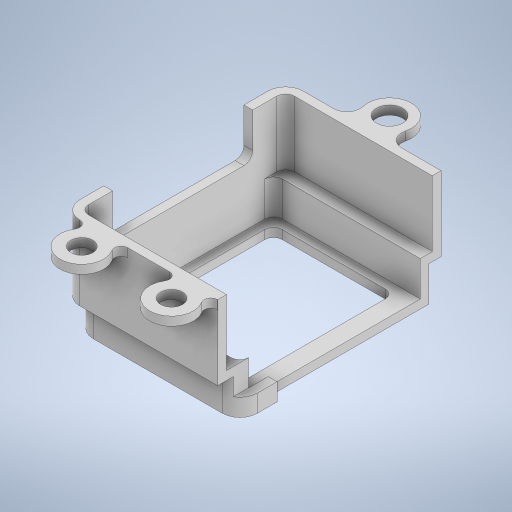
# Autodesk Inventor part: CO-1-01-motorControllersMount
Saved by Autodesk Inventor 2023 (Build 270158000, 158)
## iProperties
Created: 2023-01-24
Part Number: CO-1-01-motorControllersMount
Material: Generic
Document SubType Name: Modeling
Designer: t205b
Density: 1 g/cm^3
Appearance: Default
Author: t205b
Autodesk Inventor part; units mm, degrees
ref_plane "YZ Plane" through (0, 0, 0) normal (1, 0, 0) x (0, 1, 0)
ref_plane "XZ Plane" through (0, 0, 0) normal (0, 1, 0) x (-1, 0, 0)
sketch "Sketch1" plane through (0, 0, 0) normal (0, 1, 0) x (-1, 0, 0)
  arc A0 (31.569, 13.7227) -> (30.069, 12.2227) centre (31.569, 12.2227) ccw
  line L0 (31.569, 13.7227) -> (34.069, 13.7227)
  line L1 (34.069, 13.7227) -> (34.069, 18.9227)
  line L2 (32.069, 20.9227) -> (2.569, 20.9227)
  line L3 (34.069, -13.2773) -> (31.569, -13.2773)
  arc A1 (30.069, -11.7773) -> (31.569, -13.2773) centre (31.569, -11.7773) ccw
  arc A2 (34.069, 18.9227) -> (32.069, 20.9227) centre (32.069, 18.9227) ccw
  arc A3 (34.0195, 22.4149) -> (32.069, 23.9727) centre (32.069, 21.9727) ccw
  line L4 (32.069, 23.9727) -> (-23.931, 23.9727)
  arc A4 (-23.931, 23.9727) -> (-25.931, 21.9727) centre (-23.931, 21.9727) ccw
  line L5 (-25.931, 21.9727) -> (-25.931, -21.0273)
  arc A5 (-25.931, -21.0273) -> (-23.931, -23.0273) centre (-23.931, -21.0273) ccw
  line L6 (-23.931, -23.0273) -> (32.069, -23.0273)
  arc A6 (32.069, -23.0273) -> (33.899, -21.8341) centre (32.069, -21.0273) ccw
  arc A7 (32.069, -20.2773) -> (34.069, -18.2773) centre (32.069, -18.2773) ccw
  line L7 (32.069, -20.2773) -> (0.569, -20.2773)
  line L8 (34.069, -13.2773) -> (34.069, 13.7227)
  line L9 (0.569, -22.2773) -> (0.569, 18.9227)
  line L10 (30.069, -11.7773) -> (30.069, 12.2227)
  line L11 (34.069, -18.2773) -> (34.069, -13.2773)
  line L12 (2.569, 22.9227) -> (32.069, 22.9227)
  line L13 (0.569, -22.2773) -> (32.069, -22.2773)
  arc A8 (32.069, -22.2773) -> (36.069, -18.2773) centre (32.069, -18.2773) ccw
  line L14 (36.069, -18.2773) -> (36.069, 18.9227)
  arc A9 (2.569, 20.9227) -> (0.569, 18.9227) centre (2.569, 18.9227) ccw
  line L15 (-1.431, 14.4227) -> (-1.431, 18.9227)
  arc A10 (2.569, 22.9227) -> (-1.431, 18.9227) centre (2.569, 18.9227) ccw
  arc A11 (36.069, 18.9227) -> (32.069, 22.9227) centre (32.069, 18.9227) ccw
  line L16 (-1.431, 14.4227) -> (0.569, 14.4227)
  point P0 (0.569, 20.9227)
  dimension "d8" = 2
  dimension "d9" = 2
  dimension "d66" = 2
  dimension "d67" = 2
  dimension "d68" = 4.5
  dimension "d69" = 4
  constraints: 35 end point, 27 point on circle, 12 centre point, 8 vertical, 6 horizontal, 4 point on line, 3 tangent, 2 perpendicular, 1 collinear, 9 other
  measures "d8" distance between parallel lines of L2 L12
  measures "d9" distance between parallel lines of L7 L13
  measures "d66" radius of A9
  measures "d67" radial gap between concentric circles of A9 A10
  measures "d68" distance of L15.start L15.end
  measures "d69" radius of A11
extrude "Extrusion3" add sketch "Sketch1" against normal blind 2 contours L0 L8 L3 A1 L10 A0 | A0 L10 A1 L3 L11 A7 L7 L9 A9 L2 A2 L1 L0 | L1 A2 L2 A9 L9 L16 L15 A10 L12 A11 L14 A8 L13 L7 A7 L11 L8
ref_plane "Work Plane1" through (0, 8, 0) normal (0, 1, 0) x (1, 0, 0)
extrude "Extrusion4" add sketch "Sketch1" along normal blind 8 contours L1 A2 L2 A9 L9 L16 L15 A10 L12 A11 L14 A8 L13 L7 A7 L11 L8
sketch "Sketch2" plane through (0, 8, 0) normal (0, 1, 0) x (1, 0, 0)
  line L0 (23.931, 23.0273) -> (-32.069, 23.0273) projected
  arc A0 (-32.069, 23.0273) -> (-33.899, 21.8341) centre (-32.069, 21.0273) ccw projected
  line L1 (-32.069, -23.9727) -> (23.931, -23.9727) projected
  arc A1 (-34.0195, -22.4149) -> (-32.069, -23.9727) centre (-32.069, -21.9727) ccw projected
  arc A2 (-32.069, 23.0273) -> (-34.069, 21.0273) centre (-32.069, 21.0273) ccw
  arc A3 (-34.069, -21.9727) -> (-32.069, -23.9727) centre (-32.069, -21.9727) ccw
  line L2 (-34.069, 18.2773) -> (-34.069, 13.2773) projected
  line L3 (-34.069, 13.2773) -> (-34.069, -13.7227) projected
  line L4 (-34.069, -13.7227) -> (-34.069, -18.9227) projected
  line L5 (-34.069, -21.9727) -> (-34.069, 21.0273)
  arc A4 (-32.069, 25.0273) -> (-36.069, 21.0273) centre (-32.069, 21.0273) ccw
  line L6 (-0.569, 25.0273) -> (-32.069, 25.0273)
  line L7 (-0.569, -25.9727) -> (-32.069, -25.9727)
  line L8 (-0.569, -23.9727) -> (-0.569, -25.9727)
  line L9 (-0.569, 20.2773) -> (-0.569, 25.0273)
  line L10 (-0.569, 22.2773) -> (-0.569, 22.2773) projected
  line L11 (-32.069, 23.0273) -> (-0.569, 23.0273)
  line L12 (-32.069, -23.9727) -> (-0.569, -23.9727)
  line L13 (-32.069, -20.9227) -> (-2.569, -20.9227) projected
  line L14 (-0.569, -14.4227) -> (-0.569, 20.2773) projected
  line L15 (-0.569, 20.2773) -> (-32.069, 20.2773) projected
  arc A5 (-32.069, 20.2773) -> (-34.069, 18.2773) centre (-32.069, 18.2773) ccw projected
  line L16 (-34.069, 18.2773) -> (-34.069, -18.9227) projected
  arc A6 (-34.069, -18.9227) -> (-32.069, -20.9227) centre (-32.069, -18.9227) ccw projected
  line L17 (-32.069, 22.2773) -> (-0.569, 22.2773) projected
  line L18 (-0.569, 22.2773) -> (-0.569, 22.2773)
  arc A7 (-2.569, -20.9227) -> (-0.569, -18.9227) centre (-2.569, -18.9227) ccw projected
  line L19 (-0.569, -18.9227) -> (-0.569, -14.4227) projected
  line L20 (-0.569, -23.9727) -> (-0.569, -18.9227)
  line L21 (-36.069, 21.0273) -> (-36.069, -21.9727)
  arc A8 (-36.069, -21.9727) -> (-32.069, -25.9727) centre (-32.069, -21.9727) ccw
  point P0 (0, 0)
  point P1 (-32.069, 25.0273)
  dimension "d19" = 2
  dimension "d20" = 2
  dimension "d21" = 31.5
  dimension "d22" = 31.5
  dimension "d23" = 31.5
  constraints: 22 end point, 10 point on circle, 6 point on line, 4 centre point, 4 perpendicular, 3 tangent, 2 coincident, 2 vertical, 1 concentric, 1 horizontal, 1 parallel, 1 vertical alignment, 1 other
  measures "d19" distance between parallel lines of L0 L6
  measures "d20" distance between parallel lines of L1 L7
  measures "d21" distance of L7.start L7.end
  measures "d22" distance of L1.start L8.start
  measures "d23" distance of L6.start L6.end
extrude "Extrusion7" add sketch "Sketch2" against normal blind 2 contours L9 L15 A5 L5 A2 A0 L0 | L0 A0 A2 L5 L2 L3 L4 A3 A1 L1 L8 L7 A8 L21 A4 L6 L9 | L20 L1 A1 A3 L5 A6 L13 A7
extrude "Extrusion8" add sketch "Sketch2" along normal blind 15 contours L0 A0 A2 L5 L2 L3 L4 A3 A1 L1 L8 L7 A8 L21 A4 L6 L9
sketch "Sketch5" plane through (0, 23, 0) normal (0, 1, 0) x (1, 0, 0)
  circle A0 centre (-17.319, 30.0273) radius 5
  circle A1 centre (-17.319, 30.0273) radius 3
  arc A2 (-12.4777, 28.7773) -> (-9.573, 25.0273) centre (-9.573, 28.0273) ccw
  arc A3 (-25.0649, 25.0273) -> (-22.1602, 28.7773) centre (-25.0649, 28.0273) ccw
  line L0 (-0.569, 23.0273) -> (-0.569, 25.0273) projected
  circle A4 centre (-6.0917, -30.9727) radius 5
  circle A5 centre (-6.0917, -30.9727) radius 2.5
  arc A6 (-10.305, -28.2804) -> (-11.569, -25.9727) centre (-11.569, -27.4727) ccw
  arc A7 (-0.6145, -25.9727) -> (-1.8785, -28.2804) centre (-0.6145, -27.4727) ccw
  circle A8 centre (-26.5917, -30.9727) radius 5
  circle A9 centre (-26.5917, -30.9727) radius 2.5
  arc A10 (-30.805, -28.2804) -> (-32.069, -25.9727) centre (-32.069, -27.4727) ccw
  arc A11 (-21.1145, -25.9727) -> (-22.3785, -28.2804) centre (-21.1145, -27.4727) ccw
  line L1 (-0.569, -25.9727) -> (-0.569, -23.9727) projected
  line L2 (-0.569, 25.0273) -> (-32.069, 25.0273) projected
  line L3 (-32.069, -25.9727) -> (-0.569, -25.9727) projected
  point P0 (0, 0)
  point P1 (1.0185, -24.3852)
  point P2 (-26.5917, -25.9727)
  point P3 (-6.0917, -25.9727)
  point P4 (-17.319, 25.0273)
  dimension "d34" = 10
  dimension "d35" = 6
  dimension "d38" = 3
  dimension "d39" = 3
  dimension "d40" = 10
  dimension "d41" = 5
  dimension "d42" = 3
  dimension "d43" = 3
  dimension "d44" = 10
  dimension "d45" = 5
  dimension "d46" = 3
  dimension "d47" = 3
  dimension "d49" = 20.5
  constraints: 18 point on circle, 12 centre point, 6 tangent, 3 coincident
  measures "d34" diameter of A0
  measures "d35" diameter of A1
  measures "d38" radius of A3
  measures "d39" radius of A2
  measures "d40" diameter of A4
  measures "d41" diameter of A5
  measures "d42" diameter of A6
  measures "d43" diameter of A7
  measures "d44" diameter of A8
  measures "d45" diameter of A9
  measures "d46" diameter of A10
  measures "d47" diameter of A11
  measures "d49" distance of A4.centre A8.centre
extrude "Extrusion10" add sketch "Sketch5" against normal blind 2
sketch "Sketch6" plane through (0, -2, 0) normal (0, -1, 0) x (1, 0, 0)
  line L0 (-0.569, -22.2773) -> (-0.569, 14.4227) projected
  line L1 (-2.569, 22.9227) -> (-32.069, 22.9227) projected
  arc A0 (-32.069, 22.9227) -> (-36.069, 18.9227) centre (-32.069, 18.9227) ccw projected
  line L2 (-36.069, 18.9227) -> (-36.069, -18.2773) projected
  arc A1 (-36.069, -18.2773) -> (-32.069, -22.2773) centre (-32.069, -18.2773) ccw projected
  line L3 (-32.069, -22.2773) -> (-0.569, -22.2773) projected
  line L4 (-30.069, 18.9227) -> (-6.569, 18.9227)
  line L5 (-4.569, 16.9227) -> (-4.569, -16.2773)
  line L6 (-6.569, -18.2773) -> (-30.069, -18.2773)
  line L7 (-32.069, -16.2773) -> (-32.069, 16.9227)
  arc A2 (-6.569, -18.2773) -> (-4.569, -16.2773) centre (-6.569, -16.2773) ccw
  arc A3 (-32.069, -16.2773) -> (-30.069, -18.2773) centre (-30.069, -16.2773) ccw
  arc A4 (-30.069, 18.9227) -> (-32.069, 16.9227) centre (-30.069, 16.9227) ccw
  arc A5 (-4.569, 16.9227) -> (-6.569, 18.9227) centre (-6.569, 16.9227) ccw
  line L8 (-0.569, 14.4227) -> (1.431, 14.4227) projected
  line L9 (1.431, 14.4227) -> (1.431, 18.9227) projected
  arc A6 (1.431, 18.9227) -> (-2.569, 22.9227) centre (-2.569, 18.9227) ccw projected
  point P0 (0, 0)
  point P1 (-4.569, 18.9227)
  point P2 (-4.569, -18.2773)
  dimension "d52" = 4
  dimension "d53" = 37.2
  dimension "d54" = 27.5
  dimension "d55" = 4
  dimension "d56" = 2
  constraints: 8 end point, 8 point on circle, 8 tangent, 4 centre point, 4 point on line, 3 equal radius, 3 perpendicular
  measures "d52" distance between parallel lines of L1 L4
  measures "d53" distance of point (-4.569, 18.923) point (-4.569, -18.277)
  measures "d54" distance between parallel lines of L5 L7
  measures "d55" distance between parallel lines of L0 L5
  measures "d56" radius of A2
extrude "Extrusion11" cut sketch "Sketch6" against normal blind 2 contours L4 A5 L5 A2 L6 A3 L7 A4
sketch "Sketch7" plane through (-36.069, -2, -18.2773) normal (-1, 0, 0) x (0, 0, 1)
  line L0 (2.75, 25) -> (34.75, 25)
  line L1 (34.75, 25) -> (34.75, 17)
  line L2 (32.75, 15) -> (4.75, 15)
  line L3 (2.75, 17) -> (2.75, 25)
  arc A0 (2.75, 17) -> (4.75, 15) centre (4.75, 17) ccw
  arc A1 (32.75, 15) -> (34.75, 17) centre (32.75, 17) ccw
  point P0 (18.2773, 2)
  point P1 (40.25, 25)
  point P2 (-2.75, 25)
  point P3 (34.75, 21)
  point P4 (40.25, 8)
  dimension "d59" = 2
  dimension "d61" = 32
  dimension "d62" = 43
  constraints: 8 end point, 4 point on circle, 4 tangent, 2 centre point, 2 parallel, 1 equal radius, 1 horizontal, 1 midpoint, 1 perpendicular
  measures "d59" radius of A0
  measures "d61" distance from line of point (34.75, 21) L3
  measures "d62" distance of point (40.25, 25) point (-2.75, 25)
extrude "Extrusion12" cut sketch "Sketch7" against normal blind 6
sketch "Sketch8" plane through (0, 8, 0) normal (0, 1, 0) x (1, 0, 0)
  line L0 (-0.569, -14.4227) -> (-0.569, -18.9227) projected
  line L1 (1.431, -14.4227) -> (-0.569, -14.4227) projected
  line L2 (1.431, -18.9227) -> (1.431, -14.4227) projected
  arc A0 (-0.569, -22.3868) -> (1.431, -18.9227) centre (-2.569, -18.9227) ccw projected
  line L3 (-0.569, -23.9727) -> (-0.569, -18.9227) projected
  point P0 (0, 0)
extrude "Extrusion13" cut sketch "Sketch8" against normal blind 6
body "Solid2"
